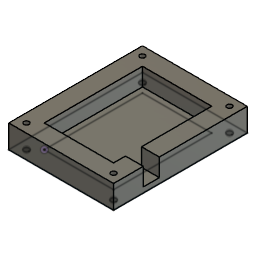
base (Autodesk Fusion 360 design; units mm, degrees)
part number: 2026-03-17-21-41-26-775
Autodesk Fusion 360 part; units mm, degrees
sketch "Sketch1" plane through (0, 0, 0) normal (0, 1, 0) x (1, 0, 0)
  line L0 (0, 0) -> (38.8, 0)
  line L1 (38.8, 0) -> (38.8, 55)
  line L2 (38.8, 55) -> (0, 55)
  line L3 (0, 55) -> (0, 0)
  line L4 (-10, 65) -> (48.8, 65)
  line L5 (48.8, 65) -> (48.8, -10)
  line L6 (48.8, -10) -> (-10, -10)
  line L7 (-10, -10) -> (-10, 65)
  circle A0 centre (-5, 60) radius 1.45
  circle A1 centre (43.8, 60) radius 1.45
  circle A2 centre (-5, -5) radius 1.45
  circle A3 centre (43.8, -5) radius 1.45
  dimension "d1" = 55
  dimension "d2" = 38.8
  dimension "d3" = 10
  dimension "d4" = 10
  dimension "d5" = 10
  dimension "d6" = 10
  dimension "d7" = 2.9
  dimension "d8" = 2.9
  dimension "d9" = 2.9
  dimension "d10" = 2.9
  dimension "d11" = 5
  dimension "d12" = 5
  dimension "d13" = 5
  dimension "d14" = 5
  dimension "d15" = 5
  dimension "d16" = 5
  dimension "d17" = 5
  dimension "d18" = 5
  constraint horizontal L0
  constraint vertical L1
  constraint horizontal L2
  constraint vertical L3
  constraint coincident L0.start L3.end
  constraint horizontal L4
  constraint vertical L5
  constraint horizontal L6
  constraint vertical L7
  measures "d1" distance of L0.start L2.end
  measures "d2" distance of L1.end L2.end
  measures "d3" distance of L2 L4
  measures "d4" distance of L3 L7
  measures "d5" distance of L1 L5
  measures "d6" distance of L0 L6
  measures "d7" diameter of A0
  measures "d8" diameter of A1
  measures "d9" diameter of A2
  measures "d10" diameter of A3
  measures "d11" distance of L4 A0.centre
  measures "d12" distance of L7 A0.centre
  measures "d13" distance of L6 A2.centre
  measures "d14" distance of L7 A2.centre
  measures "d15" distance of L6 A3.centre
  measures "d16" distance of L5 A3.centre
  measures "d17" distance of L5 A1.centre
  measures "d18" distance of L4 A1.centre
extrude "Extrude1" add sketch "Sketch1" along normal blind 3 contours L0 L1 L2 L3
extrude "Extrude2" add sketch "Sketch1" along normal blind 13
sketch "Sketch2" plane through (48.8, 0, 0) normal (1, 0, 0) x (0, 0, -1)
  line L0 (-10, 0) -> (65, 0)
  line L1 (65, 0) -> (65, 13)
  line L2 (65, 13) -> (-10, 13)
  line L3 (-10, 13) -> (-10, 0)
  line L4 (-10, 13) -> (0, 13)
  line L5 (0, 0) -> (-10, 0)
  line L6 (-10, 0) -> (-10, 13)
  line L7 (0, 13) -> (6.675, 13)
  line L8 (6.675, 13) -> (6.675, 0)
  line L9 (6.675, 0) -> (0, 0)
  line L10 (6.675, 13) -> (15.675, 13)
  line L11 (15.675, 13) -> (15.675, 3)
  line L12 (15.675, 3) -> (6.675, 3)
  line L13 (6.675, 3) -> (6.675, 13)
  line L14 (65, 0) -> (-10, 0)
  dimension "d23" = 6.675
  dimension "d24" = 9
  dimension "d25" = 3
  constraint horizontal L4
  constraint horizontal L5
  constraint vertical L6
  constraint coincident L5.start L9.end
  constraint coincident L2.end L3.start
  constraint horizontal L7
  constraint vertical L8
  constraint horizontal L9
  constraint coincident L0 L8.end
  constraint horizontal L10
  constraint vertical L11
  constraint horizontal L12
  constraint vertical L13
  measures "d23" distance of L4.end L7.end
  measures "d24" distance of L7.end L10.end
  measures "d25" distance of L12 L14
extrude "Extrude3" cut sketch "Sketch2" against normal blind 10 contours L2 L8 L10 L11 L12 L13
